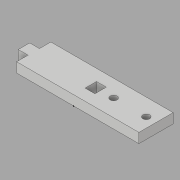
# Autodesk Inventor part: g_arm_v_1
Saved by Autodesk Inventor 2019 (Build 230136000, 136)
## iProperties
Created: 2021-11-02
Part Number: g_arm_v_1
Material: Generic
Document SubType Name: Modeling
Designer: Mohamed
Density: 1 g/cm^3
Appearance: Default
Author: Mohamed
Autodesk Inventor part; units mm, degrees
ref_plane "YZ Plane" through (0, 0, 0) normal (1, 0, 0) x (0, 1, 0)
ref_plane "XZ Plane" through (0, 0, 0) normal (0, 1, 0) x (-1, 0, 0)
ref_plane "XY Plane" through (0, 0, 0) normal (0, 0, 1) x (1, 0, 0)
sketch "Sketch1" plane through (0, 0, 0) normal (1, 0, 0) x (0, 1, 0)
  point P0 (0, 0)
sketch "Sketch2" plane through (0, 0, 0) normal (0, 1, 0) x (-1, 0, 0)
  line L0 (0, 0) -> (35, 0)
  line L1 (35, -21) -> (0, -21)
  line L2 (35, -7) -> (41, -7)
  line L3 (41, -7) -> (41, -14)
  line L4 (41, -14) -> (35, -14)
  line L5 (35, 0) -> (35, -7)
  line L6 (35, -14) -> (35, -21)
  line L7 (0, -21) -> (-40, -21)
  line L8 (-40, -21) -> (-40, 0)
  line L9 (-40, 0) -> (0, 0)
  circle A0 centre (-34, -10.5) radius 2.1
  circle A1 centre (-14, -10.5) radius 2.1
  line L10 (0, -7) -> (-6, -7)
  line L11 (-6, -7) -> (-6, -14)
  line L12 (-6, -14) -> (0, -14)
  line L13 (0, -14) -> (0, -7)
  dimension "d0" = 35
  dimension "d1" = 21
  dimension "d2" = 7
  dimension "d3" = 6
  dimension "d4" = 7
  dimension "d5" = 40
  dimension "d8" = 4.2
  dimension "d10" = 4.2
  dimension "d11" = 6
  dimension "d12" = 7
  constraints: 28 end point, 6 perpendicular, 3 horizontal, 2 centre point, 2 vertical, 1 parallel
  measures "d0" distance of L1.start L1.end
  measures "d1" distance of L0.end L1.start
  measures "d2" distance of L0.end L2.start
  measures "d3" distance of L2.start L2.end
  measures "d4" distance of L2.end L3.end
  measures "d5" distance of L1.end L7.end
  measures "d8" diameter of A0
  measures "d10" diameter of A1
  measures "d11" distance of L10.start L10.end
  measures "d12" distance of L10.end L11.end
extrude "Extrusion1" add sketch "Sketch2" along normal blind 6
body "Solid1"
